L1 (Autodesk Fusion 360 design; units mm, degrees)
part number: 2026-06-01-05-17-09-065
Autodesk Fusion 360 part; units mm, degrees
sketch "Sketch1" plane through (0, 0, 0) normal (0, 0, 1) x (1, 0, 0)
  line L0 (0, 0) -> (150, 0)
  line L1 (150, 0) -> (150, 10)
  line L2 (150, 10) -> (0, 10)
  line L3 (0, 10) -> (0, 0)
  dimension "d1" = 150
  dimension "d2" = 10
  constraint horizontal L0
  constraint vertical L1
  constraint horizontal L2
  constraint vertical L3
  constraint coincident L0.start L3.end
  measures "d1" distance of L0.start L0.end
  measures "d2" distance of L0.start L2.end
extrude "Extrude1" add sketch "Sketch1" along normal blind 10
sketch "Sketch2" plane through (0, 0, 0) normal (1, 0, 0) x (0, 1, 0)
  circle A0 centre (5, 5) radius 4
  circle A1 centre (5, 5) radius 3.5
  dimension "d5" = 8
  dimension "d6" = 7
  constraint concentric A0 A1
  measures "d5" diameter of A0
  measures "d6" diameter of A1
extrude "Extrude2" add sketch "Sketch2" against normal blind 3
sketch "Sketch3" plane through (150, 0, 0) normal (1, 0, 0) x (0, 1, 0)
  line L0 (0, 0) -> (10, 0)
  line L1 (10, 0) -> (10, 10)
  line L2 (10, 10) -> (0, 10)
  line L3 (0, 10) -> (0, 0)
  circle A0 centre (5, 5) radius 4.5
  dimension "d9" = 9
  measures "d9" diameter of A0
extrude "Extrude3" cut sketch "Sketch3" against normal blind 3 contours A0
fillet "Fillet1" radius 0.25 1 edges at (150, 0.8045, 6.6273)
sketch "Sketch4" plane through (0, 0, 0) normal (0, 0, -1) x (1, 0, 0)
  line L0 (0, 0) -> (0, -10)
  line L1 (0, -10) -> (150, -10)
  line L2 (150, -10) -> (150, 0)
  line L3 (150, 0) -> (0, 0)
  circle A0 centre (5, -5) radius 4.5
  circle A1 centre (25, -5) radius 4.5
  circle A2 centre (65, -5) radius 4.5
  circle A3 centre (45, -5) radius 4.5
  circle A4 centre (145, -5) radius 4.5
  circle A5 centre (125, -5) radius 4.5
  circle A6 centre (105, -5) radius 4.5
  circle A7 centre (85, -5) radius 4.5
  dimension "d14" = 9
  dimension "d15" = 9
  dimension "d16" = 9
  dimension "d17" = 9
  dimension "d18" = 9
  dimension "d19" = 9
  dimension "d20" = 9
  dimension "d21" = 9
  measures "d14" diameter of A0
  measures "d15" diameter of A1
  measures "d16" diameter of A3
  measures "d17" diameter of A2
  measures "d18" diameter of A7
  measures "d19" diameter of A6
  measures "d20" diameter of A5
  measures "d21" diameter of A4
extrude "Extrude4" cut sketch "Sketch4" against normal blind 30 contours A0 | A1 | A2 | A3 | A4 | A5 | A6 | A7
sketch "Sketch5" plane through (0, 10, 0) normal (0, 1, 0) x (-1, 0, 0)
  line L0 (-150, 0) -> (0, 0)
  line L1 (0, 0) -> (0, 10)
  line L2 (0, 10) -> (-150, 10)
  line L3 (-150, 10) -> (-150, 0)
  circle A0 centre (-15, 5) radius 4.5
  circle A1 centre (-35, 5) radius 4.5
  circle A2 centre (-75, 5) radius 4.5
  circle A3 centre (-55, 5) radius 4.5
  circle A4 centre (-95, 5) radius 4.5
  circle A5 centre (-115, 5) radius 4.5
  circle A6 centre (-135, 5) radius 4.5
  dimension "d24" = 9
  dimension "d25" = 9
  dimension "d26" = 9
  dimension "d27" = 9
  dimension "d28" = 9
  dimension "d29" = 9
  dimension "d30" = 9
  measures "d24" diameter of A0
  measures "d25" diameter of A1
  measures "d26" diameter of A3
  measures "d27" diameter of A2
  measures "d28" diameter of A4
  measures "d29" diameter of A5
  measures "d30" diameter of A6
extrude "Extrude5" cut sketch "Sketch5" against normal blind 30 contours A0 | A1 | A2 | A3 | A4 | A5 | A6
sketch "Sketch6" plane through (0, 0, 0) normal (0, 0, -1) x (1, 0, 0)
  line L0 (0, 0) -> (0, -10)
  line L1 (0, -10) -> (150, -10)
  line L2 (150, -10) -> (150, 0)
  line L3 (150, 0) -> (0, 0)
  circle A0 centre (145, -5) radius 4.5
  circle A1 centre (65, -5) radius 4.5
  circle A2 centre (5, -5) radius 4.5
  circle A3 centre (85, -5) radius 4.5
  circle A4 centre (125, -5) radius 4.5
  circle A5 centre (45, -5) radius 4.5
  circle A6 centre (25, -5) radius 4.5
  circle A7 centre (105, -5) radius 4.5
extrude "Extrude6" add sketch "Sketch6" against normal blind 10 contours A0
sketch "Sketch7" plane through (150, 0, 0) normal (1, 0, 0) x (0, 1, 0)
  line L0 (0, 0) -> (10, 0)
  line L1 (10, 0) -> (10, 10)
  line L2 (10, 10) -> (0, 10)
  line L3 (0, 10) -> (0, 0)
  circle A0 centre (5, 5) radius 4.75
extrude "Extrude7" cut sketch "Sketch7" against normal blind 3 contours A0
extrude "Extrude8" cut 1 faces at (147, 4.6477, 2.9844) along direction (-1, 0, 0) blind 0.5
